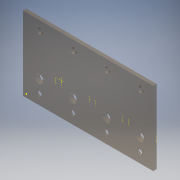
# Autodesk Inventor part: talon stack mount
Saved by Autodesk Inventor 2019 (Build 230136000, 136)
## iProperties
Created: 2019-01-16
Part Number: talon stack mount
Material: Polycarbonate, Smoke
Document SubType Name: Modeling
Designer: pctech
Density: 1.2 g/cm^3
Appearance: Polycarbonate - Smoked
Mass: 31.6682 g
Surface Area: 185.044 cm^2
Volume: 26.3901 cm^3
Author: pctech
Autodesk Inventor part; units mm, degrees
ref_plane "YZ Plane" through (0, 0, 0) normal (1, 0, 0) x (0, 1, 0)
ref_plane "XZ Plane" through (0, 0, 0) normal (0, 1, 0) x (-1, 0, 0)
ref_plane "XY Plane" through (0, 0, 0) normal (0, 0, 1) x (1, 0, 0)
sketch "Sketch1" plane through (0, 0, 0) normal (0, 0, 1) x (1, 0, 0)
  line L0 (0, 0) -> (123.19, 0)
  line L1 (123.19, 0) -> (123.19, 69.85)
  line L2 (123.19, 69.85) -> (0, 69.85)
  line L3 (0, 69.85) -> (0, 0)
  dimension "d0" = 69.85
  dimension "d1" = 123.19
  constraints: 8 end point, 2 parallel, 1 horizontal, 1 perpendicular
  measures "d0" distance of L2.end L0.start
  measures "d1" distance of L0.start L0.end
extrude "Extrusion1" add sketch "Sketch1" along normal blind 3.175
sketch "Sketch2" plane through (0, 0, 3.175) normal (0, 0, 1) x (1, 0, 0)
  line L0 (123.19, 69.85) -> (0, 69.85) projected
  line L1 (0, 69.85) -> (0, 0) projected
  point P0 (15.24, 60.071)
  point P1 (46.99, 60.071)
  point P2 (78.74, 60.071)
  point P3 (110.49, 60.071)
  dimension "d5" = 9.779
  dimension "d6" = 15.24
  dimension "d7" = 31.75
  dimension "d8" = 31.75
  dimension "d9" = 31.75
  constraints: 3 horizontal alignment
  measures "d5" distance from line of L0 point (15.24, 60.071)
  measures "d6" distance from line of L1 point (15.24, 60.071)
  measures "d7" distance of point (46.99, 60.071) point (15.24, 60.071)
  measures "d8" distance of point (78.74, 60.071) point (46.99, 60.071)
  measures "d9" distance of point (110.49, 60.071) point (78.74, 60.071)
hole "Hole1" at (15.24, 60.071, 3.175) at (46.99, 60.071, 3.175) at (78.74, 60.071, 3.175) at (110.49, 60.071, 3.175) direction (0, 0, -1) diameter 4.4958 end through all clearance for "Flat Head Machine Screw (82)" size "#8" standard "Ansi Unified Screw Threads"
sketch "Sketch3" plane through (0, 0, 3.175) normal (0, 0, 1) x (1, 0, 0)
  circle A0 centre (110.49, 60.071) radius 2.2479 projected
  circle A1 centre (46.99, 60.071) radius 2.2479 projected
  circle A2 centre (15.24, 60.071) radius 2.2479 projected
  circle A3 centre (78.74, 60.071) radius 2.2479 projected
  line L0 (0, 0) -> (123.19, 0) projected
  line L1 (123.19, 0) -> (123.19, 69.85) projected
  line L2 (123.19, 69.85) -> (0, 69.85) projected
  line L3 (0, 69.85) -> (0, 0) projected
  point P0 (15.24, 21.5392)
  point P1 (46.99, 21.5392)
  point P2 (78.74, 21.5392)
  point P3 (110.49, 21.5392)
  constraints: 3 horizontal alignment
hole "Hole2" at (15.24, 21.5392, 3.175) at (46.99, 21.5392, 3.175) at (78.74, 21.5392, 3.175) at (110.49, 21.5392, 3.175) direction (0, 0, -1) diameter 4.4958 end through all countersink diameter 8.4328 countersink angle 82 clearance for "Flat Head Machine Screw (82)" size "#8" standard "Ansi Unified Screw Threads"
sketch "Sketch4" plane through (0, 0, 0) normal (0, 0, -1) x (-1, 0, 0)
  circle A0 centre (-78.74, 21.5392) radius 2.2479 projected
  circle A1 centre (-15.24, 21.5392) radius 2.2479 projected
  circle A2 centre (-46.99, 21.5392) radius 2.2479 projected
  circle A3 centre (-110.49, 21.5392) radius 2.2479 projected
  circle A4 centre (-78.74, 60.071) radius 2.2479 projected
  circle A5 centre (-15.24, 60.071) radius 2.2479 projected
  circle A6 centre (-46.99, 60.071) radius 2.2479 projected
  circle A7 centre (-110.49, 60.071) radius 2.2479 projected
  line L0 (0, 0) -> (-123.19, 0) projected
  line L1 (0, 69.85) -> (0, 0) projected
  line L2 (-123.19, 69.85) -> (0, 69.85) projected
  line L3 (-123.19, 0) -> (-123.19, 69.85) projected
  point P0 (-110.49, 9.271)
  point P1 (-78.74, 9.271)
  point P2 (-46.99, 9.271)
  point P3 (-15.24, 9.271)
  dimension "d26" = 50.8
  constraints: 4 vertical alignment, 3 horizontal alignment
  measures "d26" distance of A5.centre point (-15.24, 9.271)
hole "Hole3" at (110.49, 9.271, 0) at (78.74, 9.271, 0) at (46.99, 9.271, 0) at (15.24, 9.271, 0) direction (0, 0, 1) diameter 4.4958 end through all countersink diameter 8.4328 countersink angle 82 clearance for "Flat Head Machine Screw (82)" size "#8" standard "Ansi Unified Screw Threads"
sketch "Sketch5" plane through (0, 0, 0) normal (0, 0, -1) x (-1, 0, 0)
  line L0 (-27.6957, 27.45) -> (-27.6957, 22.55) construction
  line L1 (-28.4154, 27.65) -> (-27.2311, 27.65) construction
  line L2 (-27.2311, 22.35) -> (-28.4154, 22.35) construction
  line L3 (-32.8311, 22.35) -> (-34.0154, 22.35) construction
  line L4 (-33.5508, 22.55) -> (-33.5508, 27.45) construction
  line L5 (-34.0154, 27.65) -> (-32.8311, 27.65) construction
  line L6 (-59.4457, 27.45) -> (-59.4457, 22.55) construction
  line L7 (-60.1654, 27.65) -> (-58.9811, 27.65) construction
  line L8 (-65.7654, 27.65) -> (-64.5811, 27.65) construction
  line L9 (-65.25, 22.55) -> (-65.25, 27.45) construction
  line L10 (-64.5811, 22.35) -> (-65.7654, 22.35) construction
  line L11 (-91.9154, 27.65) -> (-90.7311, 27.65) construction
  line L12 (-91.1957, 27.45) -> (-91.1957, 22.55) construction
  line L13 (-90.7311, 22.35) -> (-91.9154, 22.35) construction
  line L14 (-96.3311, 22.35) -> (-97.5154, 22.35) construction
  line L15 (-97.0508, 22.55) -> (-97.0508, 27.45) construction
  line L16 (-97.5154, 27.65) -> (-96.3311, 27.65) construction
  line L17 (-122.9457, 27.45) -> (-122.9457, 22.55) construction
  line L18 (-123.6654, 27.65) -> (-122.4811, 27.65) construction
  line L19 (-122.4811, 22.35) -> (-123.6654, 22.35) construction
  line L20 (-123.6654, 27.65) -> (0, 27.65) construction
  line L21 (0, 27.65) -> (0, 22.35) construction
  line L22 (0, 69.85) -> (0, 0) construction
  line L23 (-123.6654, 22.35) -> (0, 22.35) construction
  line L24 (-97.0508, 27.65) -> (-97.0508, 22.35) construction
  line L25 (-123.19, 27.396) -> (0, 27.396)
  line L26 (0, 27.396) -> (0, 22.604)
  line L27 (0, 22.604) -> (-123.19, 22.604)
  line L28 (-123.19, 22.604) -> (-123.19, 27.396)
  line L29 (0, 69.85) -> (0, 0) projected
  line L30 (-123.19, 0) -> (-123.19, 69.85) projected
  line L31 (-97.0508, 27.396) -> (-97.0508, 22.55)
  line L32 (-91.1957, 27.45) -> (-91.1957, 22.55)
  line L33 (-65.25, 27.45) -> (-65.25, 22.604)
  line L34 (-59.4457, 27.45) -> (-59.4457, 22.55)
  line L35 (-33.5508, 27.45) -> (-33.5508, 22.55)
  line L36 (-27.6957, 27.45) -> (-27.6957, 22.604)
  dimension "d34" = 0.254
  dimension "d35" = 0.254
  constraints: 28 end point, 10 point on line, 7 collinear, 2 horizontal, 2 parallel, 2 perpendicular, 1 other
  measures "d34" distance between parallel lines of L23 L27
  measures "d35" distance between parallel lines of L25 L20
equation "\"d8\" = d7"
equation "\"d9\" = d7"
equation "\"d35\" = d34"
body "Solid1"
